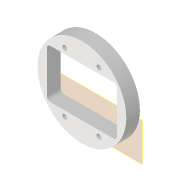
# Autodesk Inventor part: Anglerfish_spacer8mm_bottom_v0
Saved by Autodesk Inventor 2022 (Build 260153000, 153)
## iProperties
Created: 2022-09-05
Part Number: Anglerfish_spacer8mm_bottom_v0
Material: Generisch
Document SubType Name: Modeling
Designer: UC2
Density: 1 g/cm^3
Appearance: Vorgabe
Author: UC2
Autodesk Inventor part; units mm, degrees
ref_plane "YZ Plane" through (0, 0, 0) normal (1, 0, 0) x (0, 1, 0)
ref_plane "XZ Plane" through (0, 0, 0) normal (0, 1, 0) x (-1, 0, 0)
ref_plane "XY Plane" through (0, 0, 0) normal (0, 0, 1) x (1, 0, 0)
ref_plane "Arbeitsebene1" through (426.5914, 236.3923, -168.6308) normal (0, 0, -1) x (0.9997639, 0.0217278, 0)
sketch "Skizze1" plane through (426.5914, 236.3923, -168.6308) normal (0, 0, -1) x (0.9997639, 0.0217278, 0)
  circle A0 centre (-10, -17.5) radius 1.4 projected
  arc A1 (-22.2323, -12) -> (-21.7536, -14.2401) centre (-19.0971, -12.5012) ccw projected
  arc A2 (-21.7536, -14.2401) -> (-13.215, -22.3912) centre (0, 0) ccw projected
  arc A3 (-13.215, -22.3912) -> (-8.8966, -21.32) centre (-11.6012, -19.6569) ccw projected
  arc A4 (-2.8797, -22.9216) -> (-8.8966, -21.32) centre (-6.1282, -23.0224) ccw projected
  arc A5 (-2.8797, -22.9216) -> (0.3346, -25.9978) centre (0.2937, -22.8231) ccw projected
  arc A6 (0.3346, -25.9978) -> (25.1076, -6.7536) centre (0, 0) ccw projected
  arc A7 (25.1076, -6.7536) -> (24.1419, -5.4938) centre (24.1419, -6.4938) ccw projected
  line L0 (24.1419, -5.4938) -> (21.5, -5.4938) projected
  arc A8 (21.5, -5.4938) -> (20.5, -6.4938) centre (21.5, -6.4938) ccw projected
  line L1 (20.5, -6.4938) -> (20.5, -12.25) projected
  arc A9 (19.5653, -13.9427) -> (20.5, -12.25) centre (18.5, -12.25) ccw projected
  arc A10 (19.5653, -13.9427) -> (18.3317, -15.4908) centre (21.1633, -16.4816) ccw projected
  arc A11 (15.5, -17.5) -> (18.3317, -15.4908) centre (15.5, -14.5) ccw projected
  line L2 (15.5, -17.5) -> (11.4, -17.5) projected
  arc A12 (10.611, -16.2403) -> (11.4, -17.5) centre (10, -17.5) ccw projected
  line L3 (10.611, -16.2403) -> (10.611, -14.3079) projected
  arc A13 (10.611, -14.3079) -> (10.0242, -14.25) centre (10.0242, -17.25) ccw projected
  line L4 (10.0242, -14.25) -> (-18.5, -14.25) projected
  arc A14 (-20.5, -12.25) -> (-18.5, -14.25) centre (-18.5, -12.25) ccw projected
  line L5 (-20.5, -12.25) -> (-20.5, -12) projected
  line L6 (-22.2323, -12) -> (-20.5, -12) projected
  arc A15 (14.1536, 17.8908) -> (13.1449, 22.4324) centre (11.5397, 19.693) ccw projected
  arc A16 (13.1449, 22.4324) -> (-23.0651, 12) centre (0, 0) ccw projected
  line L7 (-20.5, 12) -> (-23.0651, 12) projected
  line L8 (-20.5, 12) -> (-20.5, 12.25) projected
  arc A17 (-18.5, 14.25) -> (-20.5, 12.25) centre (-18.5, 12.25) ccw projected
  line L9 (-18.5, 14.25) -> (10.0242, 14.25) projected
  arc A18 (10.0242, 14.25) -> (10.611, 14.3079) centre (10.0242, 17.25) ccw projected
  line L10 (10.611, 14.3079) -> (10.611, 16.2403) projected
  arc A19 (11.3618, 17.8248) -> (10.611, 16.2403) centre (10, 17.5) ccw projected
  line L11 (11.3618, 17.8248) -> (14.1093, 17.8248) projected
  arc A20 (14.1536, 17.8908) -> (14.1093, 17.8248) centre (16.8293, 16.046) ccw projected
  circle A21 centre (-10, 17.5) radius 1.4 projected
  circle A22 centre (10, 17.5) radius 1.4
  circle A23 centre (10, -17.5) radius 1.4
  circle A24 centre (0, 0) radius 26
  circle A25 centre (0, 0) radius 24.1513
  line L12 (-20.5, -12) -> (-20.5, 12)
  arc A26 (23.033, 12.0616) -> (19.834, 13.7401) centre (20.2203, 10.5887) ccw projected
  arc A27 (20.5, 12.25) -> (19.834, 13.7401) centre (18.5, 12.25) ccw projected
  line L13 (20.5, 12.25) -> (20.5, 7.4938) projected
  arc A28 (20.5, 7.4938) -> (21.5, 6.4938) centre (21.5, 7.4938) ccw projected
  line L14 (21.5, 6.4938) -> (23.8504, 6.4938) projected
  arc A29 (23.8504, 6.4938) -> (24.8044, 7.7936) centre (23.8504, 7.4938) ccw projected
  arc A30 (24.8044, 7.7936) -> (23.033, 12.0616) centre (0, 0) ccw projected
  line L15 (20.5, -6.4938) -> (20.5, 7.4938)
  line L16 (10.611, 14.3079) -> (19.4569, 14.3079)
  line L17 (10.0242, -14.25) -> (19.4993, -14.25)
  point P0 (-431.6269, 227.0676)
  point P1 (14.6734, 19.1827)
  point P2 (19.9142, 13.6642)
  point P3 (19.9142, -13.6642)
  point P4 (18.1109, -15.9775)
  point P5 (13.1449, 22.4324)
  point P6 (-21.7536, -14.2401)
  point P7 (-13.215, -22.3912)
  point P8 (0.3346, -25.9978)
  point P9 (25.1076, -6.7536)
  point P10 (11.4, -17.5)
  constraints: 8 end point, 4 centre point, 3 coincident, 3 concentric, 3 point on circle, 1 collinear, 1 horizontal, 1 parallel, 1 perpendicular
extrude "Extrusion1" add sketch "Skizze1" along normal blind 8 contours L6 A25 A14 A3 A2 A1 | A1 A24 L7 A25 L6 | A25 L7 L12 L6 | L6 L5 A14 A25 | A3 A25 A5 A24 | A16 A15 A25 A17 L7 | L17 A10 A11 A25 L2 A23 L3 A13 | A25 A17 L8 L7 | A25 A14 L4 A13 L3 A12 L2 A11 A5 A4 A3 | A3 A4 A5 A25 | A5 A25 A11 A9 L0 A7 A6 | A24 A26 A25 A15 | A7 L0 A25 L14 A29 A24 | A25 L16 L10 A22 L11 A20 A15 | A15 A20 L11 A19 L10 A18 L9 A17 A25 | A24 A29 L14 A25 A27 A26 | A25 A11 | A11 A10 L17 A25 | A25 A9 L1 A8 L0 | L0 A8 L15 A28 L14 A25 | L14 A28 L13 A27 A25
